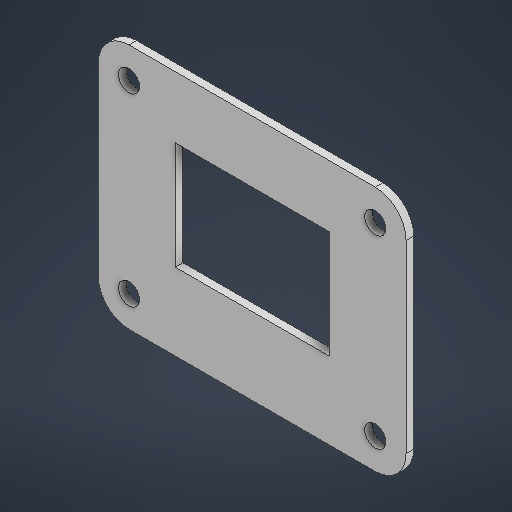
# Autodesk Inventor part: leaf
Saved by Autodesk Inventor 2026.1 (Build 301233000, 233)
## iProperties
Created: 2025-08-09
Part Number: leaf
Material: Generic
Document SubType Name: Modeling
Designer: roejo
Density: 1 g/cm^3
Appearance: Default
Author: roejo
Autodesk Inventor part; units mm, degrees
ref_plane "YZ Plane" through (0, 0, 0) normal (1, 0, 0) x (0, 1, 0)
ref_plane "XZ Plane" through (0, 0, 0) normal (0, 1, 0) x (-1, 0, 0)
ref_plane "XY Plane" through (0, 0, 0) normal (0, 0, 1) x (1, 0, 0)
sketch "Sketch1" plane through (0, 0, 0) normal (0, 0, 1) x (1, 0, 0)
  circle A0 centre (-25.609, -18.9943) radius 2.1844
  circle A1 centre (25.191, -18.9943) radius 2.1844
  arc A2 (-31.959, -18.9943) -> (-25.609, -25.3443) centre (-25.609, -18.9943) ccw
  arc A3 (25.191, -25.3443) -> (31.541, -18.9943) centre (25.191, -18.9943) ccw
  circle A4 centre (-25.609, 19.1057) radius 2.1844
  circle A5 centre (25.191, 19.1057) radius 2.1844
  arc A6 (31.541, 19.1057) -> (25.191, 25.4557) centre (25.191, 19.1057) ccw
  arc A7 (-25.609, 25.4557) -> (-31.959, 19.1057) centre (-25.609, 19.1057) ccw
  line L0 (31.541, 19.1057) -> (31.541, -18.9943)
  line L1 (25.191, 25.4557) -> (-25.609, 25.4557)
  line L2 (-31.959, 19.1057) -> (-31.959, -18.9943)
  line L3 (25.191, -25.3443) -> (-25.609, -25.3443)
  line L4 (15.666, 12.7557) -> (-16.084, 12.7557)
  line L5 (-16.084, 12.7557) -> (-16.084, -9.4693)
  line L6 (-16.084, -9.4693) -> (15.666, -9.4693)
  line L7 (15.666, -9.4693) -> (15.666, 12.7557)
  line L8 (-25.609, -18.9943) -> (-25.609, -12.6443)
  point P0 (0, 0)
  point P1 (25.191, 0.0557)
  dimension "d0" = 12.7
  dimension "d1" = 12.7
  dimension "d2" = 4.3688
  dimension "d3" = 4.3688
  dimension "d4" = 12.7
  dimension "d5" = 12.7
  dimension "d6" = 31.75
  dimension "d7" = 22.225
  dimension "d8" = 9.525
  dimension "d9" = 12.7
  constraints: 18 end point, 8 centre point, 8 point on circle, 7 tangent, 4 coincident, 2 parallel, 1 horizontal, 1 perpendicular, 1 vertical
  measures "d0" diameter of A2
  measures "d1" diameter of A3
  measures "d2" diameter of A4
  measures "d3" diameter of A5
  measures "d4" diameter of A6
  measures "d5" diameter of A7
  measures "d6" distance of L6.end L5.end
  measures "d7" distance of L5.end L4.end
  measures "d8" distance from line of point (25.191, 0.056) L7
  measures "d9" distance between parallel lines of L1 L4
extrude "Extrusion1" add sketch "Sketch1" along normal blind 1.5875
body "Solid1"
